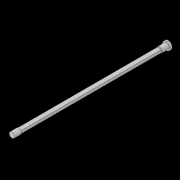
# Autodesk Inventor part: MotorMount_Part
Saved by Autodesk Inventor 2017 (Build 210142000, 142)
## iProperties
Created: 2017-01-13
Part Number: MotorMount_Part
Material: Generic
Document SubType Name: Modeling
Designer: David Kopala
Density: 1 g/cm^3
Appearance: Default
Author: David Kopala
Autodesk Inventor part; units mm, degrees
ref_plane "YZ Plane" through (0, 0, 0) normal (1, 0, 0) x (0, 1, 0)
ref_plane "XZ Plane" through (0, 0, 0) normal (0, 1, 0) x (-1, 0, 0)
ref_plane "XY Plane" through (0, 0, 0) normal (0, 0, 1) x (1, 0, 0)
sketch "Sketch1" plane through (0, 0, 0) normal (0, 0, 1) x (1, 0, 0)
  line L0 (0, 0) -> (7.62, 0)
  line L1 (7.62, 0) -> (7.62, 5.08)
  line L2 (7.62, 5.08) -> (0, 5.08)
  line L3 (0, 5.08) -> (0, 0)
  dimension "d0" = 7.62
  dimension "d1" = 5.08
  constraints: 8 end point, 2 parallel, 1 horizontal, 1 perpendicular
  measures "d0" distance of L2.end L1.end
  measures "d1" distance of L1.end L0.end
extrude "Extrusion1" add sketch "Sketch1" along normal blind 259.8166
sketch "Sketch2" plane through (0, 0, 259.8166) normal (0, 0, 1) x (1, 0, 0)
  circle A0 centre (3.8115, 2.54) radius 5.08
  line L0 (7.62, 5.08) -> (0, 5.08) projected
  line L1 (7.62, 0) -> (7.62, 5.08) projected
  point P0 (0, 0)
  dimension "d4" = 10.16
  dimension "d5" = 2.54
  dimension "d6" = 3.8085
  constraints: 1 centre point
  measures "d4" diameter of A0
  measures "d5" distance from line of A0.centre L0
  measures "d6" distance from line of L1 A0.centre
extrude "Extrusion2" add sketch "Sketch2" along normal blind 12.7
sketch "Sketch3" plane through (0, 0, 0) normal (0, 0, -1) x (-1, 0, 0)
  circle A0 centre (-3.8115, 2.54) radius 5.08
  circle A1 centre (-3.8115, 2.54) radius 5.08 projected
  point P0 (0, 0)
  dimension "d9" = 10.16
  constraints: 1 centre point, 1 concentric
  measures "d9" diameter of A0
extrude "Extrusion3" add sketch "Sketch3" along normal blind 12.7
sketch "Sketch4" plane through (3.8115, 2.54, -12.7) normal (0, 0, -1) x (-1, 0, 0)
  circle A0 centre (0, 0) radius 7.62
  point P0 (3.8115, -2.54)
  dimension "d12" = 15.24
  constraints: 1 centre point
  measures "d12" diameter of A0
extrude "Extrusion4" add sketch "Sketch4" along normal blind 3.175
body "Solid1"
